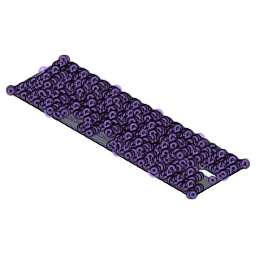
top_layout v3 (Autodesk Fusion 360 design; units mm, degrees)
Autodesk Fusion 360 part; units mm, degrees
(part 1 of 8)
sketch "Sketch2" plane through (0, 0, 0) normal (0, 0, 1) x (1, 0, 0)
  line L0 (124.062, 16.7831) -> (124.062, 15.7827)
  line L1 (124.062, 15.7827) -> (123.263, 15.7827)
  line L2 (123.263, 15.7827) -> (123.263, 12.6848)
  line L3 (123.263, 12.6848) -> (124.062, 12.6848)
  line L4 (124.062, 12.6848) -> (124.062, 12.0826)
  line L5 (124.062, 12.0826) -> (84.4381, 12.0826)
  line L6 (84.4381, 12.0826) -> (84.4381, 15.3128)
  line L7 (84.4381, 15.3128) -> (77.687, 15.3128)
  line L8 (77.687, 15.3128) -> (77.687, 12.0826)
  line L9 (77.687, 12.0826) -> (76.8629, 12.0826)
  line L10 (76.8629, 12.0826) -> (76.8629, 9.2838)
  line L11 (76.8629, 9.2838) -> (77.687, 9.2838)
  line L12 (77.687, 9.2838) -> (77.687, 3.0138)
  line L13 (77.687, 3.0138) -> (79.412, 3.0138)
  line L14 (79.412, 3.0138) -> (79.412, 1.8135)
  line L15 (79.412, 1.8135) -> (82.7126, 1.8135)
  line L16 (82.7126, 1.8135) -> (82.7126, 3.0138)
  line L17 (82.7126, 3.0138) -> (84.4381, 3.0138)
  line L18 (84.4381, 3.0138) -> (84.4381, 7.4841)
  line L19 (84.4381, 7.4841) -> (124.062, 7.4841)
  line L20 (124.062, 7.4841) -> (124.062, 6.8833)
  line L21 (124.062, 6.8833) -> (123.263, 6.8833)
  line L22 (123.263, 6.8833) -> (123.263, 3.7827)
  line L23 (123.263, 3.7827) -> (124.062, 3.7827)
  line L24 (124.062, 3.7827) -> (124.062, 2.7836)
  line L25 (124.062, 2.7836) -> (138.063, 2.7836)
  line L26 (138.063, 2.7836) -> (138.063, 3.7827)
  line L27 (138.063, 3.7827) -> (138.862, 3.7827)
  line L28 (138.862, 3.7827) -> (138.862, 6.8833)
  line L29 (138.862, 6.8833) -> (138.063, 6.8833)
  line L30 (138.063, 6.8833) -> (138.063, 7.4841)
  line L31 (138.063, 7.4841) -> (177.687, 7.4841)
  line L32 (177.687, 7.4841) -> (177.687, 3.0138)
  line L33 (177.687, 3.0138) -> (179.412, 3.0138)
  line L34 (179.412, 3.0138) -> (179.412, 1.8135)
  line L35 (179.412, 1.8135) -> (182.713, 1.8135)
  line L36 (182.713, 1.8135) -> (182.713, 3.0138)
  line L37 (182.713, 3.0138) -> (184.438, 3.0138)
  line L38 (184.438, 3.0138) -> (184.438, 9.2838)
  line L39 (184.438, 9.2838) -> (185.262, 9.2838)
  line L40 (185.262, 9.2838) -> (185.262, 12.0826)
  line L41 (185.262, 12.0826) -> (184.438, 12.0826)
  line L42 (184.438, 12.0826) -> (184.438, 15.3128)
  line L43 (184.438, 15.3128) -> (177.687, 15.3128)
  line L44 (177.687, 15.3128) -> (177.687, 12.0826)
  line L45 (177.687, 12.0826) -> (138.063, 12.0826)
  line L46 (138.063, 12.0826) -> (138.063, 12.6848)
  line L47 (138.063, 12.6848) -> (138.862, 12.6848)
  line L48 (138.862, 12.6848) -> (138.862, 15.7827)
  line L49 (138.862, 15.7827) -> (138.063, 15.7827)
  line L50 (138.063, 15.7827) -> (138.063, 16.7831)
  line L51 (138.063, 16.7831) -> (124.062, 16.7831)
  line L52 (5.0009, 16.7831) -> (5.0009, 15.7827)
  line L53 (5.0009, 15.7827) -> (4.2003, 15.7827)
  line L54 (4.2003, 15.7827) -> (4.2003, 12.6848)
  line L55 (4.2003, 12.6848) -> (5.0009, 12.6848)
  line L56 (5.0009, 12.6848) -> (5.0009, 6.8833)
  line L57 (5.0009, 6.8833) -> (4.2003, 6.8833)
  line L58 (4.2003, 6.8833) -> (4.2003, 3.7827)
  line L59 (4.2003, 3.7827) -> (5.0009, 3.7827)
  line L60 (5.0009, 3.7827) -> (5.0009, 2.7836)
  line L61 (5.0009, 2.7836) -> (19.0004, 2.7836)
  line L62 (19.0004, 2.7836) -> (19.0004, 3.7827)
  line L63 (19.0004, 3.7827) -> (19.801, 3.7827)
  line L64 (19.801, 3.7827) -> (19.801, 6.8833)
  line L65 (19.801, 6.8833) -> (19.0004, 6.8833)
  line L66 (19.0004, 6.8833) -> (19.0004, 12.6848)
  line L67 (19.0004, 12.6848) -> (19.801, 12.6848)
  line L68 (19.801, 12.6848) -> (19.801, 15.7827)
  line L69 (19.801, 15.7827) -> (19.0004, 15.7827)
  line L70 (19.0004, 15.7827) -> (19.0004, 16.7831)
  line L71 (19.0004, 16.7831) -> (5.0009, 16.7831)
  line L72 (28.812, 16.7831) -> (28.812, 15.7827)
  line L73 (28.812, 15.7827) -> (28.0128, 15.7827)
  line L74 (28.0128, 15.7827) -> (28.0128, 12.6848)
  line L75 (28.0128, 12.6848) -> (28.812, 12.6848)
  line L76 (28.812, 12.6848) -> (28.812, 6.8833)
  line L77 (28.812, 6.8833) -> (28.0128, 6.8833)
  line L78 (28.0128, 6.8833) -> (28.0128, 3.7827)
  line L79 (28.0128, 3.7827) -> (28.812, 3.7827)
  line L80 (28.812, 3.7827) -> (28.812, 2.7836)
  line L81 (28.812, 2.7836) -> (42.8128, 2.7836)
  line L82 (42.8128, 2.7836) -> (42.8128, 3.7827)
  line L83 (42.8128, 3.7827) -> (43.6122, 3.7827)
  line L84 (43.6122, 3.7827) -> (43.6122, 6.8833)
  line L85 (43.6122, 6.8833) -> (42.8128, 6.8833)
  line L86 (42.8128, 6.8833) -> (42.8128, 12.6848)
  line L87 (42.8128, 12.6848) -> (43.6122, 12.6848)
  line L88 (43.6122, 12.6848) -> (43.6122, 15.7827)
  line L89 (43.6122, 15.7827) -> (42.8128, 15.7827)
  line L90 (42.8128, 15.7827) -> (42.8128, 16.7831)
  line L91 (42.8128, 16.7831) -> (28.812, 16.7831)
  line L92 (52.626, 16.7831) -> (52.626, 15.7827)
  line L93 (52.626, 15.7827) -> (51.8252, 15.7827)
  line L94 (51.8252, 15.7827) -> (51.8252, 12.6848)
  line L95 (51.8252, 12.6848) -> (52.626, 12.6848)
  line L96 (52.626, 12.6848) -> (52.626, 6.8833)
  line L97 (52.626, 6.8833) -> (51.8252, 6.8833)
  line L98 (51.8252, 6.8833) -> (51.8252, 3.7827)
  line L99 (51.8252, 3.7827) -> (52.626, 3.7827)
  line L100 (52.626, 3.7827) -> (52.626, 2.7836)
  line L101 (52.626, 2.7836) -> (66.6253, 2.7836)
  line L102 (66.6253, 2.7836) -> (66.6253, 3.7827)
  line L103 (66.6253, 3.7827) -> (67.4261, 3.7827)
  line L104 (67.4261, 3.7827) -> (67.4261, 6.8833)
  line L105 (67.4261, 6.8833) -> (66.6253, 6.8833)
  line L106 (66.6253, 6.8833) -> (66.6253, 12.6848)
  line L107 (66.6253, 12.6848) -> (67.4261, 12.6848)
  line L108 (67.4261, 12.6848) -> (67.4261, 15.7827)
  line L109 (67.4261, 15.7827) -> (66.6253, 15.7827)
  line L110 (66.6253, 15.7827) -> (66.6253, 16.7831)
  line L111 (66.6253, 16.7831) -> (52.626, 16.7831)
  line L112 (195.501, 16.7831) -> (195.501, 15.7827)
  line L113 (195.501, 15.7827) -> (194.7, 15.7827)
  line L114 (194.7, 15.7827) -> (194.7, 12.6848)
  line L115 (194.7, 12.6848) -> (195.501, 12.6848)
  line L116 (195.501, 12.6848) -> (195.501, 6.8833)
  line L117 (195.501, 6.8833) -> (194.7, 6.8833)
  line L118 (194.7, 6.8833) -> (194.7, 3.7827)
  line L119 (194.7, 3.7827) -> (195.501, 3.7827)
  line L120 (195.501, 3.7827) -> (195.501, 2.7836)
  line L121 (195.501, 2.7836) -> (209.5, 2.7836)
  line L122 (209.5, 2.7836) -> (209.5, 3.7827)
  line L123 (209.5, 3.7827) -> (210.301, 3.7827)
  line L124 (210.301, 3.7827) -> (210.301, 6.8833)
  line L125 (210.301, 6.8833) -> (209.5, 6.8833)
  line L126 (209.5, 6.8833) -> (209.5, 12.6848)
  line L127 (209.5, 12.6848) -> (210.301, 12.6848)
  line L128 (210.301, 12.6848) -> (210.301, 15.7827)
  line L129 (210.301, 15.7827) -> (209.5, 15.7827)
  line L130 (209.5, 15.7827) -> (209.5, 16.7831)
  line L131 (209.5, 16.7831) -> (195.501, 16.7831)
  line L132 (219.312, 16.7831) -> (219.312, 15.7827)
  line L133 (219.312, 15.7827) -> (218.513, 15.7827)
  line L134 (218.513, 15.7827) -> (218.513, 12.6848)
  line L135 (218.513, 12.6848) -> (219.312, 12.6848)
  line L136 (219.312, 12.6848) -> (219.312, 6.8833)
  line L137 (219.312, 6.8833) -> (218.513, 6.8833)
  line L138 (218.513, 6.8833) -> (218.513, 3.7827)
  line L139 (218.513, 3.7827) -> (219.312, 3.7827)
  line L140 (219.312, 3.7827) -> (219.312, 2.7836)
  line L141 (219.312, 2.7836) -> (233.313, 2.7836)
  line L142 (233.313, 2.7836) -> (233.313, 3.7827)
  line L143 (233.313, 3.7827) -> (234.112, 3.7827)
  line L144 (234.112, 3.7827) -> (234.112, 6.8833)
  line L145 (234.112, 6.8833) -> (233.313, 6.8833)
  line L146 (233.313, 6.8833) -> (233.313, 12.6848)
  line L147 (233.313, 12.6848) -> (234.112, 12.6848)
  line L148 (234.112, 12.6848) -> (234.112, 15.7827)
  line L149 (234.112, 15.7827) -> (233.313, 15.7827)
  line L150 (233.313, 15.7827) -> (233.313, 16.7831)
  line L151 (233.313, 16.7831) -> (219.312, 16.7831)
  line L152 (243.126, 16.7831) -> (243.126, 15.7827)
  line L153 (243.126, 15.7827) -> (242.325, 15.7827)
  line L154 (242.325, 15.7827) -> (242.325, 12.6848)
  line L155 (242.325, 12.6848) -> (243.126, 12.6848)
  line L156 (243.126, 12.6848) -> (243.126, 6.8833)
  line L157 (243.126, 6.8833) -> (242.325, 6.8833)
  line L158 (242.325, 6.8833) -> (242.325, 3.7827)
  line L159 (242.325, 3.7827) -> (243.126, 3.7827)
  line L160 (243.126, 3.7827) -> (243.126, 2.7836)
  line L161 (243.126, 2.7836) -> (257.125, 2.7836)
  line L162 (257.125, 2.7836) -> (257.125, 3.7827)
  line L163 (257.125, 3.7827) -> (257.926, 3.7827)
  line L164 (257.926, 3.7827) -> (257.926, 6.8833)
  line L165 (257.926, 6.8833) -> (257.125, 6.8833)
  line L166 (257.125, 6.8833) -> (257.125, 12.6848)
  line L167 (257.125, 12.6848) -> (257.926, 12.6848)
  line L168 (257.926, 12.6848) -> (257.926, 15.7827)
  line L169 (257.926, 15.7827) -> (257.125, 15.7827)
  line L170 (257.125, 15.7827) -> (257.125, 16.7831)
  line L171 (257.125, 16.7831) -> (243.126, 16.7831)
  line L172 (274.082, 16.7831) -> (274.082, 15.7827)
  line L173 (274.082, 15.7827) -> (273.281, 15.7827)
  line L174 (273.281, 15.7827) -> (273.281, 12.6848)
  line L175 (273.281, 12.6848) -> (274.082, 12.6848)
  line L176 (274.082, 12.6848) -> (274.082, 6.8833)
  line L177 (274.082, 6.8833) -> (273.281, 6.8833)
  line L178 (273.281, 6.8833) -> (273.281, 3.7827)
  line L179 (273.281, 3.7827) -> (274.082, 3.7827)
  line L180 (274.082, 3.7827) -> (274.082, 2.7836)
  line L181 (274.082, 2.7836) -> (288.082, 2.7836)
  line L182 (288.082, 2.7836) -> (288.082, 3.7827)
  line L183 (288.082, 3.7827) -> (288.881, 3.7827)
  line L184 (288.881, 3.7827) -> (288.881, 6.8833)
  line L185 (288.881, 6.8833) -> (288.082, 6.8833)
  line L186 (288.082, 6.8833) -> (288.082, 12.6848)
  line L187 (288.082, 12.6848) -> (288.881, 12.6848)
  line L188 (288.881, 12.6848) -> (288.881, 15.7827)
  line L189 (288.881, 15.7827) -> (288.082, 15.7827)
  line L190 (288.082, 15.7827) -> (288.082, 16.7831)
  line L191 (288.082, 16.7831) -> (274.082, 16.7831)
  line L192 (293.132, 16.7831) -> (293.132, 15.7827)
  line L193 (293.132, 15.7827) -> (292.331, 15.7827)
  line L194 (292.331, 15.7827) -> (292.331, 12.6848)
  line L195 (292.331, 12.6848) -> (293.132, 12.6848)
  line L196 (293.132, 12.6848) -> (293.132, 6.8833)
  line L197 (293.132, 6.8833) -> (292.331, 6.8833)
  line L198 (292.331, 6.8833) -> (292.331, 3.7827)
  line L199 (292.331, 3.7827) -> (293.132, 3.7827)
  line L200 (293.132, 3.7827) -> (293.132, 2.7836)
  line L201 (293.132, 2.7836) -> (307.132, 2.7836)
  line L202 (307.132, 2.7836) -> (307.132, 3.7827)
  line L203 (307.132, 3.7827) -> (307.931, 3.7827)
  line L204 (307.931, 3.7827) -> (307.931, 6.8833)
  line L205 (307.931, 6.8833) -> (307.132, 6.8833)
  line L206 (307.132, 6.8833) -> (307.132, 12.6848)
  line L207 (307.132, 12.6848) -> (307.931, 12.6848)
  line L208 (307.931, 12.6848) -> (307.931, 15.7827)
  line L209 (307.931, 15.7827) -> (307.132, 15.7827)
  line L210 (307.132, 15.7827) -> (307.132, 16.7831)
  line L211 (307.132, 16.7831) -> (293.132, 16.7831)
  line L212 (312.182, 16.7831) -> (312.182, 15.7827)
  line L213 (312.182, 15.7827) -> (311.381, 15.7827)
  line L214 (311.381, 15.7827) -> (311.381, 12.6848)
  line L215 (311.381, 12.6848) -> (312.182, 12.6848)
  line L216 (312.182, 12.6848) -> (312.182, 6.8833)
  line L217 (312.182, 6.8833) -> (311.381, 6.8833)
  line L218 (311.381, 6.8833) -> (311.381, 3.7827)
  line L219 (311.381, 3.7827) -> (312.182, 3.7827)
  line L220 (312.182, 3.7827) -> (312.182, 2.7836)
  line L221 (312.182, 2.7836) -> (326.182, 2.7836)
  line L222 (326.182, 2.7836) -> (326.182, 3.7827)
  line L223 (326.182, 3.7827) -> (326.981, 3.7827)
  line L224 (326.981, 3.7827) -> (326.981, 6.8833)
  line L225 (326.981, 6.8833) -> (326.182, 6.8833)
  line L226 (326.182, 6.8833) -> (326.182, 12.6848)
  line L227 (326.182, 12.6848) -> (326.981, 12.6848)
  line L228 (326.981, 12.6848) -> (326.981, 15.7827)
  line L229 (326.981, 15.7827) -> (326.182, 15.7827)
  line L230 (326.182, 15.7827) -> (326.182, 16.7831)
  line L231 (326.182, 16.7831) -> (312.182, 16.7831)
  line L232 (14.5259, 35.833) -> (14.5259, 34.8327)
  line L233 (14.5259, 34.8327) -> (13.7253, 34.8327)
  line L234 (13.7253, 34.8327) -> (13.7253, 31.7348)
  line L235 (13.7253, 31.7348) -> (14.5259, 31.7348)
  line L236 (14.5259, 31.7348) -> (14.5259, 31.1326)
  line L237 (14.5259, 31.1326) -> (13.0004, 31.1326)
  line L238 (13.0004, 31.1326) -> (13.0004, 34.3628)
  line L239 (13.0004, 34.3628) -> (6.2508, 34.3628)
  line L240 (6.2508, 34.3628) -> (6.2508, 31.1326)
  line L241 (6.2508, 31.1326) -> (5.4253, 31.1326)
  line L242 (5.4253, 31.1326) -> (5.4253, 28.3338)
  line L243 (5.4253, 28.3338) -> (6.2508, 28.3338)
  line L244 (6.2508, 28.3338) -> (6.2508, 22.0638)
  line L245 (6.2508, 22.0638) -> (7.9761, 22.0638)
  line L246 (7.9761, 22.0638) -> (7.9761, 20.8635)
  line L247 (7.9761, 20.8635) -> (11.2751, 20.8635)
  line L248 (11.2751, 20.8635) -> (11.2751, 22.0638)
  line L249 (11.2751, 22.0638) -> (13.0004, 22.0638)
  line L250 (13.0004, 22.0638) -> (13.0004, 26.5327)
  line L251 (13.0004, 26.5327) -> (14.5259, 26.5327)
  line L252 (14.5259, 26.5327) -> (14.5259, 25.9333)
  line L253 (14.5259, 25.9333) -> (13.7253, 25.9333)
  line L254 (13.7253, 25.9333) -> (13.7253, 22.8327)
  line L255 (13.7253, 22.8327) -> (14.5259, 22.8327)
  line L256 (14.5259, 22.8327) -> (14.5259, 21.8336)
  line L257 (14.5259, 21.8336) -> (28.5254, 21.8336)
  line L258 (28.5254, 21.8336) -> (28.5254, 22.8327)
  line L259 (28.5254, 22.8327) -> (29.326, 22.8327)
  line L260 (29.326, 22.8327) -> (29.326, 25.9333)
  line L261 (29.326, 25.9333) -> (28.5254, 25.9333)
  line L262 (28.5254, 25.9333) -> (28.5254, 26.5327)
  line L263 (28.5254, 26.5327) -> (30.0509, 26.5327)
  line L264 (30.0509, 26.5327) -> (30.0509, 22.0638)
  line L265 (30.0509, 22.0638) -> (31.7748, 22.0638)
  line L266 (31.7748, 22.0638) -> (31.7748, 20.8635)
  line L267 (31.7748, 20.8635) -> (35.0752, 20.8635)
  line L268 (35.0752, 20.8635) -> (35.0752, 22.0638)
  line L269 (35.0752, 22.0638) -> (36.8004, 22.0638)
  line L270 (36.8004, 22.0638) -> (36.8004, 28.3338)
  line L271 (36.8004, 28.3338) -> (37.6259, 28.3338)
  line L272 (37.6259, 28.3338) -> (37.6259, 31.1326)
  line L273 (37.6259, 31.1326) -> (36.8004, 31.1326)
  line L274 (36.8004, 31.1326) -> (36.8004, 34.3628)
  line L275 (36.8004, 34.3628) -> (30.0509, 34.3628)
  line L276 (30.0509, 34.3628) -> (30.0509, 31.1326)
  line L277 (30.0509, 31.1326) -> (28.5254, 31.1326)
  line L278 (28.5254, 31.1326) -> (28.5254, 31.7348)
  line L279 (28.5254, 31.7348) -> (29.326, 31.7348)
  line L280 (29.326, 31.7348) -> (29.326, 34.8327)
  line L281 (29.326, 34.8327) -> (28.5254, 34.8327)
  line L282 (28.5254, 34.8327) -> (28.5254, 35.833)
  line L283 (28.5254, 35.833) -> (14.5259, 35.833)
  line L284 (252.65, 35.833) -> (252.65, 34.8327)
  line L285 (252.65, 34.8327) -> (251.849, 34.8327)
  line L286 (251.849, 34.8327) -> (251.849, 31.7348)
  line L287 (251.849, 31.7348) -> (252.65, 31.7348)
  line L288 (252.65, 31.7348) -> (252.65, 31.1326)
  line L289 (252.65, 31.1326) -> (251.126, 31.1326)
  line L290 (251.126, 31.1326) -> (251.126, 34.3628)
  line L291 (251.126, 34.3628) -> (244.376, 34.3628)
  line L292 (244.376, 34.3628) -> (244.376, 31.1326)
  line L293 (244.376, 31.1326) -> (243.55, 31.1326)
  line L294 (243.55, 31.1326) -> (243.55, 28.3338)
  line L295 (243.55, 28.3338) -> (244.376, 28.3338)
  line L296 (244.376, 28.3338) -> (244.376, 22.0638)
  line L297 (244.376, 22.0638) -> (246.101, 22.0638)
  line L298 (246.101, 22.0638) -> (246.101, 20.8635)
  line L299 (246.101, 20.8635) -> (249.4, 20.8635)
  line L300 (249.4, 20.8635) -> (249.4, 22.0638)
  line L301 (249.4, 22.0638) -> (251.126, 22.0638)
  line L302 (251.126, 22.0638) -> (251.126, 26.5327)
  line L303 (251.126, 26.5327) -> (252.65, 26.5327)
  line L304 (252.65, 26.5327) -> (252.65, 25.9333)
  line L305 (252.65, 25.9333) -> (251.849, 25.9333)
  line L306 (251.849, 25.9333) -> (251.849, 22.8327)
  line L307 (251.849, 22.8327) -> (252.65, 22.8327)
  line L308 (252.65, 22.8327) -> (252.65, 21.8336)
  line L309 (252.65, 21.8336) -> (266.65, 21.8336)
  line L310 (266.65, 21.8336) -> (266.65, 22.8327)
  line L311 (266.65, 22.8327) -> (267.451, 22.8327)
  line L312 (267.451, 22.8327) -> (267.451, 25.9333)
  line L313 (267.451, 25.9333) -> (266.65, 25.9333)
  line L314 (266.65, 25.9333) -> (266.65, 26.5327)
  line L315 (266.65, 26.5327) -> (268.176, 26.5327)
  line L316 (268.176, 26.5327) -> (268.176, 22.0638)
  line L317 (268.176, 22.0638) -> (269.9, 22.0638)
  line L318 (269.9, 22.0638) -> (269.9, 20.8635)
  line L319 (269.9, 20.8635) -> (273.2, 20.8635)
  line L320 (273.2, 20.8635) -> (273.2, 22.0638)
  line L321 (273.2, 22.0638) -> (274.925, 22.0638)
  line L322 (274.925, 22.0638) -> (274.925, 28.3338)
  line L323 (274.925, 28.3338) -> (275.751, 28.3338)
  line L324 (275.751, 28.3338) -> (275.751, 31.1326)
  line L325 (275.751, 31.1326) -> (274.925, 31.1326)
  line L326 (274.925, 31.1326) -> (274.925, 34.3628)
  line L327 (274.925, 34.3628) -> (268.176, 34.3628)
  line L328 (268.176, 34.3628) -> (268.176, 31.1326)
  line L329 (268.176, 31.1326) -> (266.65, 31.1326)
  line L330 (266.65, 31.1326) -> (266.65, 31.7348)
  line L331 (266.65, 31.7348) -> (267.451, 31.7348)
  line L332 (267.451, 31.7348) -> (267.451, 34.8327)
  line L333 (267.451, 34.8327) -> (266.65, 34.8327)
  line L334 (266.65, 34.8327) -> (266.65, 35.833)
  line L335 (266.65, 35.833) -> (252.65, 35.833)
  line L336 (45.4822, 35.833) -> (45.4822, 34.8327)
  line L337 (45.4822, 34.8327) -> (44.6814, 34.8327)
  line L338 (44.6814, 34.8327) -> (44.6814, 31.7348)
  line L339 (44.6814, 31.7348) -> (45.4822, 31.7348)
  line L340 (45.4822, 31.7348) -> (45.4822, 25.9333)
  line L341 (45.4822, 25.9333) -> (44.6814, 25.9333)
  line L342 (44.6814, 25.9333) -> (44.6814, 22.8327)
  line L343 (44.6814, 22.8327) -> (45.4822, 22.8327)
  line L344 (45.4822, 22.8327) -> (45.4822, 21.8336)
  line L345 (45.4822, 21.8336) -> (59.4815, 21.8336)
  line L346 (59.4815, 21.8336) -> (59.4815, 22.8327)
  line L347 (59.4815, 22.8327) -> (60.2809, 22.8327)
  line L348 (60.2809, 22.8327) -> (60.2809, 25.9333)
  line L349 (60.2809, 25.9333) -> (59.4815, 25.9333)
  line L350 (59.4815, 25.9333) -> (59.4815, 31.7348)
  line L351 (59.4815, 31.7348) -> (60.2809, 31.7348)
  line L352 (60.2809, 31.7348) -> (60.2809, 34.8327)
  line L353 (60.2809, 34.8327) -> (59.4815, 34.8327)
  line L354 (59.4815, 34.8327) -> (59.4815, 35.833)
  line L355 (59.4815, 35.833) -> (45.4822, 35.833)
  line L356 (64.5322, 35.833) -> (64.5322, 34.8327)
  line L357 (64.5322, 34.8327) -> (63.7314, 34.8327)
  line L358 (63.7314, 34.8327) -> (63.7314, 31.7348)
  line L359 (63.7314, 31.7348) -> (64.5322, 31.7348)
  line L360 (64.5322, 31.7348) -> (64.5322, 25.9333)
  line L361 (64.5322, 25.9333) -> (63.7314, 25.9333)
  line L362 (63.7314, 25.9333) -> (63.7314, 22.8327)
  line L363 (63.7314, 22.8327) -> (64.5322, 22.8327)
  line L364 (64.5322, 22.8327) -> (64.5322, 21.8336)
  line L365 (64.5322, 21.8336) -> (78.5315, 21.8336)
  line L366 (78.5315, 21.8336) -> (78.5315, 22.8327)
  line L367 (78.5315, 22.8327) -> (79.3309, 22.8327)
  line L368 (79.3309, 22.8327) -> (79.3309, 25.9333)
  line L369 (79.3309, 25.9333) -> (78.5315, 25.9333)
  line L370 (78.5315, 25.9333) -> (78.5315, 31.7348)
  line L371 (78.5315, 31.7348) -> (79.3309, 31.7348)
  line L372 (79.3309, 31.7348) -> (79.3309, 34.8327)
  line L373 (79.3309, 34.8327) -> (78.5315, 34.8327)
  line L374 (78.5315, 34.8327) -> (78.5315, 35.833)
  line L375 (78.5315, 35.833) -> (64.5322, 35.833)
  line L376 (83.5822, 35.833) -> (83.5822, 34.8327)
  line L377 (83.5822, 34.8327) -> (82.7814, 34.8327)
  line L378 (82.7814, 34.8327) -> (82.7814, 31.7348)
  line L379 (82.7814, 31.7348) -> (83.5822, 31.7348)
  line L380 (83.5822, 31.7348) -> (83.5822, 25.9333)
  line L381 (83.5822, 25.9333) -> (82.7814, 25.9333)
  line L382 (82.7814, 25.9333) -> (82.7814, 22.8327)
  line L383 (82.7814, 22.8327) -> (83.5822, 22.8327)
  line L384 (83.5822, 22.8327) -> (83.5822, 21.8336)
  line L385 (83.5822, 21.8336) -> (97.5815, 21.8336)
  line L386 (97.5815, 21.8336) -> (97.5815, 22.8327)
  line L387 (97.5815, 22.8327) -> (98.3809, 22.8327)
  line L388 (98.3809, 22.8327) -> (98.3809, 25.9333)
  line L389 (98.3809, 25.9333) -> (97.5815, 25.9333)
  line L390 (97.5815, 25.9333) -> (97.5815, 31.7348)
  line L391 (97.5815, 31.7348) -> (98.3809, 31.7348)
  line L392 (98.3809, 31.7348) -> (98.3809, 34.8327)
  line L393 (98.3809, 34.8327) -> (97.5815, 34.8327)
  line L394 (97.5815, 34.8327) -> (97.5815, 35.833)
  line L395 (97.5815, 35.833) -> (83.5822, 35.833)
  line L396 (102.632, 35.833) -> (102.632, 34.8327)
  line L397 (102.632, 34.8327) -> (101.831, 34.8327)
  line L398 (101.831, 34.8327) -> (101.831, 31.7348)
  line L399 (101.831, 31.7348) -> (102.632, 31.7348)
  line L400 (102.632, 31.7348) -> (102.632, 25.9333)
  line L401 (102.632, 25.9333) -> (101.831, 25.9333)
  line L402 (101.831, 25.9333) -> (101.831, 22.8327)
  line L403 (101.831, 22.8327) -> (102.632, 22.8327)
  line L404 (102.632, 22.8327) -> (102.632, 21.8336)
  line L405 (102.632, 21.8336) -> (116.632, 21.8336)
  line L406 (116.632, 21.8336) -> (116.632, 22.8327)
  line L407 (116.632, 22.8327) -> (117.431, 22.8327)
  line L408 (117.431, 22.8327) -> (117.431, 25.9333)
  line L409 (117.431, 25.9333) -> (116.632, 25.9333)
  line L410 (116.632, 25.9333) -> (116.632, 31.7348)
  line L411 (116.632, 31.7348) -> (117.431, 31.7348)
  line L412 (117.431, 31.7348) -> (117.431, 34.8327)
  line L413 (117.431, 34.8327) -> (116.632, 34.8327)
  line L414 (116.632, 34.8327) -> (116.632, 35.833)
  line L415 (116.632, 35.833) -> (102.632, 35.833)
  line L416 (121.682, 35.833) -> (121.682, 34.8327)
  line L417 (121.682, 34.8327) -> (120.881, 34.8327)
  line L418 (120.881, 34.8327) -> (120.881, 31.7348)
  line L419 (120.881, 31.7348) -> (121.682, 31.7348)
  line L420 (121.682, 31.7348) -> (121.682, 25.9333)
  line L421 (121.682, 25.9333) -> (120.881, 25.9333)
  line L422 (120.881, 25.9333) -> (120.881, 22.8327)
  line L423 (120.881, 22.8327) -> (121.682, 22.8327)
  line L424 (121.682, 22.8327) -> (121.682, 21.8336)
  line L425 (121.682, 21.8336) -> (135.682, 21.8336)
  line L426 (135.682, 21.8336) -> (135.682, 22.8327)
  line L427 (135.682, 22.8327) -> (136.481, 22.8327)
  line L428 (136.481, 22.8327) -> (136.481, 25.9333)
  line L429 (136.481, 25.9333) -> (135.682, 25.9333)
  line L430 (135.682, 25.9333) -> (135.682, 31.7348)
  line L431 (135.682, 31.7348) -> (136.481, 31.7348)
  line L432 (136.481, 31.7348) -> (136.481, 34.8327)
  line L433 (136.481, 34.8327) -> (135.682, 34.8327)
  line L434 (135.682, 34.8327) -> (135.682, 35.833)
  line L435 (135.682, 35.833) -> (121.682, 35.833)
  line L436 (140.732, 35.833) -> (140.732, 34.8327)
  line L437 (140.732, 34.8327) -> (139.931, 34.8327)
  line L438 (139.931, 34.8327) -> (139.931, 31.7348)
  line L439 (139.931, 31.7348) -> (140.732, 31.7348)
  line L440 (140.732, 31.7348) -> (140.732, 25.9333)
  line L441 (140.732, 25.9333) -> (139.931, 25.9333)
  line L442 (139.931, 25.9333) -> (139.931, 22.8327)
  line L443 (139.931, 22.8327) -> (140.732, 22.8327)
  line L444 (140.732, 22.8327) -> (140.732, 21.8336)
  line L445 (140.732, 21.8336) -> (154.732, 21.8336)
  line L446 (154.732, 21.8336) -> (154.732, 22.8327)
  line L447 (154.732, 22.8327) -> (155.531, 22.8327)
  line L448 (155.531, 22.8327) -> (155.531, 25.9333)
  line L449 (155.531, 25.9333) -> (154.732, 25.9333)
  line L450 (154.732, 25.9333) -> (154.732, 31.7348)
  line L451 (154.732, 31.7348) -> (155.531, 31.7348)
  line L452 (155.531, 31.7348) -> (155.531, 34.8327)
  line L453 (155.531, 34.8327) -> (154.732, 34.8327)
  line L454 (154.732, 34.8327) -> (154.732, 35.833)
  line L455 (154.732, 35.833) -> (140.732, 35.833)
  line L456 (159.782, 35.833) -> (159.782, 34.8327)
  line L457 (159.782, 34.8327) -> (158.981, 34.8327)
  line L458 (158.981, 34.8327) -> (158.981, 31.7348)
  line L459 (158.981, 31.7348) -> (159.782, 31.7348)
  line L460 (159.782, 31.7348) -> (159.782, 25.9333)
  line L461 (159.782, 25.9333) -> (158.981, 25.9333)
  line L462 (158.981, 25.9333) -> (158.981, 22.8327)
  line L463 (158.981, 22.8327) -> (159.782, 22.8327)
  line L464 (159.782, 22.8327) -> (159.782, 21.8336)
  line L465 (159.782, 21.8336) -> (173.782, 21.8336)
  line L466 (173.782, 21.8336) -> (173.782, 22.8327)
  line L467 (173.782, 22.8327) -> (174.581, 22.8327)
  line L468 (174.581, 22.8327) -> (174.581, 25.9333)
  line L469 (174.581, 25.9333) -> (173.782, 25.9333)
  line L470 (173.782, 25.9333) -> (173.782, 31.7348)
  line L471 (173.782, 31.7348) -> (174.581, 31.7348)
  line L472 (174.581, 31.7348) -> (174.581, 34.8327)
  line L473 (174.581, 34.8327) -> (173.782, 34.8327)
  line L474 (173.782, 34.8327) -> (173.782, 35.833)
  line L475 (173.782, 35.833) -> (159.782, 35.833)
  line L476 (178.832, 35.833) -> (178.832, 34.8327)
  line L477 (178.832, 34.8327) -> (178.031, 34.8327)
  line L478 (178.031, 34.8327) -> (178.031, 31.7348)
  line L479 (178.031, 31.7348) -> (178.832, 31.7348)
  line L480 (178.832, 31.7348) -> (178.832, 25.9333)
  line L481 (178.832, 25.9333) -> (178.031, 25.9333)
  line L482 (178.031, 25.9333) -> (178.031, 22.8327)
  line L483 (178.031, 22.8327) -> (178.832, 22.8327)
  line L484 (178.832, 22.8327) -> (178.832, 21.8336)
  line L485 (178.832, 21.8336) -> (192.832, 21.8336)
  line L486 (192.832, 21.8336) -> (192.832, 22.8327)
  line L487 (192.832, 22.8327) -> (193.631, 22.8327)
  line L488 (193.631, 22.8327) -> (193.631, 25.9333)
  line L489 (193.631, 25.9333) -> (192.832, 25.9333)
  line L490 (192.832, 25.9333) -> (192.832, 31.7348)
  line L491 (192.832, 31.7348) -> (193.631, 31.7348)
  line L492 (193.631, 31.7348) -> (193.631, 34.8327)
  line L493 (193.631, 34.8327) -> (192.832, 34.8327)
  line L494 (192.832, 34.8327) -> (192.832, 35.833)
  line L495 (192.832, 35.833) -> (178.832, 35.833)
  line L496 (197.882, 35.833) -> (197.882, 34.8327)
  line L497 (197.882, 34.8327) -> (197.081, 34.8327)
  line L498 (197.081, 34.8327) -> (197.081, 31.7348)
  line L499 (197.081, 31.7348) -> (197.882, 31.7348)
  line L500 (197.882, 31.7348) -> (197.882, 25.9333)
  line L501 (197.882, 25.9333) -> (197.081, 25.9333)
  line L502 (197.081, 25.9333) -> (197.081, 22.8327)
  line L503 (197.081, 22.8327) -> (197.882, 22.8327)
  line L504 (197.882, 22.8327) -> (197.882, 21.8336)
  line L505 (197.882, 21.8336) -> (211.882, 21.8336)
  line L506 (211.882, 21.8336) -> (211.882, 22.8327)
  line L507 (211.882, 22.8327) -> (212.681, 22.8327)
  line L508 (212.681, 22.8327) -> (212.681, 25.9333)
  line L509 (212.681, 25.9333) -> (211.882, 25.9333)
  line L510 (211.882, 25.9333) -> (211.882, 31.7348)
  line L511 (211.882, 31.7348) -> (212.681, 31.7348)
  line L512 (212.681, 31.7348) -> (212.681, 34.8327)
  line L513 (212.681, 34.8327) -> (211.882, 34.8327)
  line L514 (211.882, 34.8327) -> (211.882, 35.833)
  line L515 (211.882, 35.833) -> (197.882, 35.833)
  line L516 (216.932, 35.833) -> (216.932, 34.8327)
  line L517 (216.932, 34.8327) -> (216.131, 34.8327)
  line L518 (216.131, 34.8327) -> (216.131, 31.7348)
  line L519 (216.131, 31.7348) -> (216.932, 31.7348)
  line L520 (216.932, 31.7348) -> (216.932, 25.9333)
  line L521 (216.932, 25.9333) -> (216.131, 25.9333)
  line L522 (216.131, 25.9333) -> (216.131, 22.8327)
  line L523 (216.131, 22.8327) -> (216.932, 22.8327)
  line L524 (216.932, 22.8327) -> (216.932, 21.8336)
  line L525 (216.932, 21.8336) -> (230.932, 21.8336)
  line L526 (230.932, 21.8336) -> (230.932, 22.8327)
  line L527 (230.932, 22.8327) -> (231.731, 22.8327)
  line L528 (231.731, 22.8327) -> (231.731, 25.9333)
  line L529 (231.731, 25.9333) -> (230.932, 25.9333)
  line L530 (230.932, 25.9333) -> (230.932, 31.7348)
  line L531 (230.932, 31.7348) -> (231.731, 31.7348)
  line L532 (231.731, 31.7348) -> (231.731, 34.8327)
  line L533 (231.731, 34.8327) -> (230.932, 34.8327)
  line L534 (230.932, 34.8327) -> (230.932, 35.833)
  line L535 (230.932, 35.833) -> (216.932, 35.833)
  line L536 (293.132, 35.833) -> (293.132, 34.8327)
  line L537 (293.132, 34.8327) -> (292.331, 34.8327)
  line L538 (292.331, 34.8327) -> (292.331, 31.7348)
  line L539 (292.331, 31.7348) -> (293.132, 31.7348)
  line L540 (293.132, 31.7348) -> (293.132, 25.9333)
  line L541 (293.132, 25.9333) -> (292.331, 25.9333)
  line L542 (292.331, 25.9333) -> (292.331, 22.8327)
  line L543 (292.331, 22.8327) -> (293.132, 22.8327)
  line L544 (293.132, 22.8327) -> (293.132, 21.8336)
  line L545 (293.132, 21.8336) -> (307.132, 21.8336)
  line L546 (307.132, 21.8336) -> (307.132, 22.8327)
  line L547 (307.132, 22.8327) -> (307.931, 22.8327)
  line L548 (307.931, 22.8327) -> (307.931, 25.9333)
  line L549 (307.931, 25.9333) -> (307.132, 25.9333)
  line L550 (307.132, 25.9333) -> (307.132, 31.7348)
  line L551 (307.132, 31.7348) -> (307.931, 31.7348)
  line L552 (307.931, 31.7348) -> (307.931, 34.8327)
  line L553 (307.931, 34.8327) -> (307.132, 34.8327)
  line L554 (307.132, 34.8327) -> (307.132, 35.833)
  line L555 (307.132, 35.833) -> (293.132, 35.833)
  line L556 (257.412, 54.8831) -> (257.412, 53.8826)
  line L557 (257.412, 53.8826) -> (256.611, 53.8826)
  line L558 (256.611, 53.8826) -> (256.611, 50.7834)
  line L559 (256.611, 50.7834) -> (257.412, 50.7834)
  line L560 (257.412, 50.7834) -> (257.412, 50.1826)
  line L561 (257.412, 50.1826) -> (255.888, 50.1826)
  line L562 (255.888, 50.1826) -> (255.888, 53.4127)
  line L563 (255.888, 53.4127) -> (249.137, 53.4127)
  line L564 (249.137, 53.4127) -> (249.137, 50.1826)
  line L565 (249.137, 50.1826) -> (248.313, 50.1826)
  line L566 (248.313, 50.1826) -> (248.313, 47.3837)
  line L567 (248.313, 47.3837) -> (249.137, 47.3837)
  line L568 (249.137, 47.3837) -> (249.137, 41.1138)
  line L569 (249.137, 41.1138) -> (250.862, 41.1138)
  line L570 (250.862, 41.1138) -> (250.862, 39.9136)
  line L571 (250.862, 39.9136) -> (254.161, 39.9136)
  line L572 (254.161, 39.9136) -> (254.161, 41.1138)
  line L573 (254.161, 41.1138) -> (255.888, 41.1138)
  line L574 (255.888, 41.1138) -> (255.888, 45.5828)
  line L575 (255.888, 45.5828) -> (257.412, 45.5828)
  line L576 (257.412, 45.5828) -> (257.412, 44.9834)
  line L577 (257.412, 44.9834) -> (256.611, 44.9834)
  line L578 (256.611, 44.9834) -> (256.611, 41.8828)
  line L579 (256.611, 41.8828) -> (257.412, 41.8828)
  line L580 (257.412, 41.8828) -> (257.412, 40.8838)
  line L581 (257.412, 40.8838) -> (271.413, 40.8838)
  line L582 (271.413, 40.8838) -> (271.413, 41.8828)
  line L583 (271.413, 41.8828) -> (272.212, 41.8828)
  line L584 (272.212, 41.8828) -> (272.212, 44.9834)
  line L585 (272.212, 44.9834) -> (271.413, 44.9834)
  line L586 (271.413, 44.9834) -> (271.413, 45.5828)
  line L587 (271.413, 45.5828) -> (272.937, 45.5828)
  line L588 (272.937, 45.5828) -> (272.937, 41.1138)
  line L589 (272.937, 41.1138) -> (274.662, 41.1138)
  line L590 (274.662, 41.1138) -> (274.662, 39.9136)
  line L591 (274.662, 39.9136) -> (277.963, 39.9136)
  line L592 (277.963, 39.9136) -> (277.963, 41.1138)
  line L593 (277.963, 41.1138) -> (279.688, 41.1138)
  line L594 (279.688, 41.1138) -> (279.688, 47.3837)
  line L595 (279.688, 47.3837) -> (280.512, 47.3837)
  line L596 (280.512, 47.3837) -> (280.512, 50.1826)
  line L597 (280.512, 50.1826) -> (279.688, 50.1826)
  line L598 (279.688, 50.1826) -> (279.688, 53.4127)
  line L599 (279.688, 53.4127) -> (272.937, 53.4127)
  line L600 (272.937, 53.4127) -> (272.937, 50.1826)
  line L601 (272.937, 50.1826) -> (271.413, 50.1826)
  line L602 (271.413, 50.1826) -> (271.413, 50.7834)
  line L603 (271.413, 50.7834) -> (272.212, 50.7834)
  line L604 (272.212, 50.7834) -> (272.212, 53.8826)
  line L605 (272.212, 53.8826) -> (271.413, 53.8826)
  line L606 (271.413, 53.8826) -> (271.413, 54.8831)
  line L607 (271.413, 54.8831) -> (257.412, 54.8831)
  line L608 (9.762, 54.8831) -> (9.762, 53.8826)
  line L609 (9.762, 53.8826) -> (8.9628, 53.8826)
  line L610 (8.9628, 53.8826) -> (8.9628, 50.7834)
  line L611 (8.9628, 50.7834) -> (9.762, 50.7834)
  line L612 (9.762, 50.7834) -> (9.762, 44.9834)
  line L613 (9.762, 44.9834) -> (8.9628, 44.9834)
  line L614 (8.9628, 44.9834) -> (8.9628, 41.8828)
  line L615 (8.9628, 41.8828) -> (9.762, 41.8828)
  line L616 (9.762, 41.8828) -> (9.762, 40.8838)
  line L617 (9.762, 40.8838) -> (23.7629, 40.8838)
  line L618 (23.7629, 40.8838) -> (23.7629, 41.8828)
  line L619 (23.7629, 41.8828) -> (24.5622, 41.8828)
  line L620 (24.5622, 41.8828) -> (24.5622, 44.9834)
  line L621 (24.5622, 44.9834) -> (23.7629, 44.9834)
  line L622 (23.7629, 44.9834) -> (23.7629, 50.7834)
  line L623 (23.7629, 50.7834) -> (24.5622, 50.7834)
  line L624 (24.5622, 50.7834) -> (24.5622, 53.8826)
  line L625 (24.5622, 53.8826) -> (23.7629, 53.8826)
  line L626 (23.7629, 53.8826) -> (23.7629, 54.8831)
  line L627 (23.7629, 54.8831) -> (9.762, 54.8831)
  line L628 (35.9572, 54.8831) -> (35.9572, 53.8826)
  line L629 (35.9572, 53.8826) -> (35.1565, 53.8826)
  line L630 (35.1565, 53.8826) -> (35.1565, 50.7834)
  line L631 (35.1565, 50.7834) -> (35.9572, 50.7834)
  line L632 (35.9572, 50.7834) -> (35.9572, 44.9834)
  line L633 (35.9572, 44.9834) -> (35.1565, 44.9834)
  line L634 (35.1565, 44.9834) -> (35.1565, 41.8828)
  line L635 (35.1565, 41.8828) -> (35.9572, 41.8828)
  line L636 (35.9572, 41.8828) -> (35.9572, 40.8838)
  line L637 (35.9572, 40.8838) -> (49.9565, 40.8838)
  line L638 (49.9565, 40.8838) -> (49.9565, 41.8828)
  line L639 (49.9565, 41.8828) -> (50.7559, 41.8828)
  line L640 (50.7559, 41.8828) -> (50.7559, 44.9834)
  line L641 (50.7559, 44.9834) -> (49.9565, 44.9834)
  line L642 (49.9565, 44.9834) -> (49.9565, 50.7834)
  line L643 (49.9565, 50.7834) -> (50.7559, 50.7834)
  line L644 (50.7559, 50.7834) -> (50.7559, 53.8826)
  line L645 (50.7559, 53.8826) -> (49.9565, 53.8826)
  line L646 (49.9565, 53.8826) -> (49.9565, 54.8831)
  line L647 (49.9565, 54.8831) -> (35.9572, 54.8831)
  line L648 (55.0072, 54.8831) -> (55.0072, 53.8826)
  line L649 (55.0072, 53.8826) -> (54.2064, 53.8826)
  line L650 (54.2064, 53.8826) -> (54.2064, 50.7834)
  line L651 (54.2064, 50.7834) -> (55.0072, 50.7834)
  line L652 (55.0072, 50.7834) -> (55.0072, 44.9834)
  line L653 (55.0072, 44.9834) -> (54.2064, 44.9834)
  line L654 (54.2064, 44.9834) -> (54.2064, 41.8828)
  line L655 (54.2064, 41.8828) -> (55.0072, 41.8828)
  line L656 (55.0072, 41.8828) -> (55.0072, 40.8838)
  line L657 (55.0072, 40.8838) -> (69.0065, 40.8838)
  line L658 (69.0065, 40.8838) -> (69.0065, 41.8828)
  line L659 (69.0065, 41.8828) -> (69.8059, 41.8828)
  line L660 (69.8059, 41.8828) -> (69.8059, 44.9834)
  line L661 (69.8059, 44.9834) -> (69.0065, 44.9834)
  line L662 (69.0065, 44.9834) -> (69.0065, 50.7834)
  line L663 (69.0065, 50.7834) -> (69.8059, 50.7834)
  line L664 (69.8059, 50.7834) -> (69.8059, 53.8826)
  line L665 (69.8059, 53.8826) -> (69.0065, 53.8826)
  line L666 (69.0065, 53.8826) -> (69.0065, 54.8831)
  line L667 (69.0065, 54.8831) -> (55.0072, 54.8831)
  line L668 (74.0572, 54.8831) -> (74.0572, 53.8826)
  line L669 (74.0572, 53.8826) -> (73.2564, 53.8826)
  line L670 (73.2564, 53.8826) -> (73.2564, 50.7834)
  line L671 (73.2564, 50.7834) -> (74.0572, 50.7834)
  line L672 (74.0572, 50.7834) -> (74.0572, 44.9834)
  line L673 (74.0572, 44.9834) -> (73.2564, 44.9834)
  line L674 (73.2564, 44.9834) -> (73.2564, 41.8828)
  line L675 (73.2564, 41.8828) -> (74.0572, 41.8828)
  line L676 (74.0572, 41.8828) -> (74.0572, 40.8838)
  line L677 (74.0572, 40.8838) -> (88.0565, 40.8838)
  line L678 (88.0565, 40.8838) -> (88.0565, 41.8828)
  line L679 (88.0565, 41.8828) -> (88.8559, 41.8828)
  line L680 (88.8559, 41.8828) -> (88.8559, 44.9834)
  line L681 (88.8559, 44.9834) -> (88.0565, 44.9834)
  line L682 (88.0565, 44.9834) -> (88.0565, 50.7834)
  line L683 (88.0565, 50.7834) -> (88.8559, 50.7834)
  line L684 (88.8559, 50.7834) -> (88.8559, 53.8826)
  line L685 (88.8559, 53.8826) -> (88.0565, 53.8826)
  line L686 (88.0565, 53.8826) -> (88.0565, 54.8831)
  line L687 (88.0565, 54.8831) -> (74.0572, 54.8831)
  line L688 (93.1072, 54.8831) -> (93.1072, 53.8826)
  line L689 (93.1072, 53.8826) -> (92.3064, 53.8826)
  line L690 (92.3064, 53.8826) -> (92.3064, 50.7834)
  line L691 (92.3064, 50.7834) -> (93.1072, 50.7834)
  line L692 (93.1072, 50.7834) -> (93.1072, 44.9834)
  line L693 (93.1072, 44.9834) -> (92.3064, 44.9834)
  line L694 (92.3064, 44.9834) -> (92.3064, 41.8828)
  line L695 (92.3064, 41.8828) -> (93.1072, 41.8828)
  line L696 (93.1072, 41.8828) -> (93.1072, 40.8838)
  line L697 (93.1072, 40.8838) -> (107.107, 40.8838)
  line L698 (107.107, 40.8838) -> (107.107, 41.8828)
  line L699 (107.107, 41.8828) -> (107.906, 41.8828)
  line L700 (107.906, 41.8828) -> (107.906, 44.9834)
  line L701 (107.906, 44.9834) -> (107.107, 44.9834)
  line L702 (107.107, 44.9834) -> (107.107, 50.7834)
  line L703 (107.107, 50.7834) -> (107.906, 50.7834)
  line L704 (107.906, 50.7834) -> (107.906, 53.8826)
  line L705 (107.906, 53.8826) -> (107.107, 53.8826)
  line L706 (107.107, 53.8826) -> (107.107, 54.8831)
  line L707 (107.107, 54.8831) -> (93.1072, 54.8831)
  line L708 (112.157, 54.8831) -> (112.157, 53.8826)
  line L709 (112.157, 53.8826) -> (111.356, 53.8826)
  line L710 (111.356, 53.8826) -> (111.356, 50.7834)
  line L711 (111.356, 50.7834) -> (112.157, 50.7834)
  line L712 (112.157, 50.7834) -> (112.157, 44.9834)
  line L713 (112.157, 44.9834) -> (111.356, 44.9834)
  line L714 (111.356, 44.9834) -> (111.356, 41.8828)
  line L715 (111.356, 41.8828) -> (112.157, 41.8828)
  line L716 (112.157, 41.8828) -> (112.157, 40.8838)
  line L717 (112.157, 40.8838) -> (126.157, 40.8838)
  line L718 (126.157, 40.8838) -> (126.157, 41.8828)
  line L719 (126.157, 41.8828) -> (126.956, 41.8828)
  line L720 (126.956, 41.8828) -> (126.956, 44.9834)
  line L721 (126.956, 44.9834) -> (126.157, 44.9834)
  line L722 (126.157, 44.9834) -> (126.157, 50.7834)
  line L723 (126.157, 50.7834) -> (126.956, 50.7834)
  line L724 (126.956, 50.7834) -> (126.956, 53.8826)
  line L725 (126.956, 53.8826) -> (126.157, 53.8826)
  line L726 (126.157, 53.8826) -> (126.157, 54.8831)
  line L727 (126.157, 54.8831) -> (112.157, 54.8831)
  line L728 (131.207, 54.8831) -> (131.207, 53.8826)
  line L729 (131.207, 53.8826) -> (130.406, 53.8826)
  line L730 (130.406, 53.8826) -> (130.406, 50.7834)
  line L731 (130.406, 50.7834) -> (131.207, 50.7834)
  line L732 (131.207, 50.7834) -> (131.207, 44.9834)
  line L733 (131.207, 44.9834) -> (130.406, 44.9834)
  line L734 (130.406, 44.9834) -> (130.406, 41.8828)
  line L735 (130.406, 41.8828) -> (131.207, 41.8828)
  line L736 (131.207, 41.8828) -> (131.207, 40.8838)
  line L737 (131.207, 40.8838) -> (145.207, 40.8838)
  line L738 (145.207, 40.8838) -> (145.207, 41.8828)
  line L739 (145.207, 41.8828) -> (146.006, 41.8828)
  line L740 (146.006, 41.8828) -> (146.006, 44.9834)
  line L741 (146.006, 44.9834) -> (145.207, 44.9834)
  line L742 (145.207, 44.9834) -> (145.207, 50.7834)
  line L743 (145.207, 50.7834) -> (146.006, 50.7834)
  line L744 (146.006, 50.7834) -> (146.006, 53.8826)
  line L745 (146.006, 53.8826) -> (145.207, 53.8826)
  line L746 (145.207, 53.8826) -> (145.207, 54.8831)
  line L747 (145.207, 54.8831) -> (131.207, 54.8831)
  line L748 (150.257, 54.8831) -> (150.257, 53.8826)
  line L749 (150.257, 53.8826) -> (149.456, 53.8826)
  line L750 (149.456, 53.8826) -> (149.456, 50.7834)
  line L751 (149.456, 50.7834) -> (150.257, 50.7834)
  line L752 (150.257, 50.7834) -> (150.257, 44.9834)
  line L753 (150.257, 44.9834) -> (149.456, 44.9834)
  line L754 (149.456, 44.9834) -> (149.456, 41.8828)
  line L755 (149.456, 41.8828) -> (150.257, 41.8828)
  line L756 (150.257, 41.8828) -> (150.257, 40.8838)
  line L757 (150.257, 40.8838) -> (164.257, 40.8838)
  line L758 (164.257, 40.8838) -> (164.257, 41.8828)
  line L759 (164.257, 41.8828) -> (165.056, 41.8828)
  line L760 (165.056, 41.8828) -> (165.056, 44.9834)
  line L761 (165.056, 44.9834) -> (164.257, 44.9834)
  line L762 (164.257, 44.9834) -> (164.257, 50.7834)
  line L763 (164.257, 50.7834) -> (165.056, 50.7834)
  line L764 (165.056, 50.7834) -> (165.056, 53.8826)
  line L765 (165.056, 53.8826) -> (164.257, 53.8826)
  line L766 (164.257, 53.8826) -> (164.257, 54.8831)
  line L767 (164.257, 54.8831) -> (150.257, 54.8831)
  line L768 (169.307, 54.8831) -> (169.307, 53.8826)
  line L769 (169.307, 53.8826) -> (168.506, 53.8826)
  line L770 (168.506, 53.8826) -> (168.506, 50.7834)
  line L771 (168.506, 50.7834) -> (169.307, 50.7834)
  line L772 (169.307, 50.7834) -> (169.307, 44.9834)
  line L773 (169.307, 44.9834) -> (168.506, 44.9834)
  line L774 (168.506, 44.9834) -> (168.506, 41.8828)
  line L775 (168.506, 41.8828) -> (169.307, 41.8828)
  line L776 (169.307, 41.8828) -> (169.307, 40.8838)
  line L777 (169.307, 40.8838) -> (183.307, 40.8838)
  line L778 (183.307, 40.8838) -> (183.307, 41.8828)
  line L779 (183.307, 41.8828) -> (184.106, 41.8828)
  line L780 (184.106, 41.8828) -> (184.106, 44.9834)
  line L781 (184.106, 44.9834) -> (183.307, 44.9834)
  line L782 (183.307, 44.9834) -> (183.307, 50.7834)
  line L783 (183.307, 50.7834) -> (184.106, 50.7834)
  line L784 (184.106, 50.7834) -> (184.106, 53.8826)
  line L785 (184.106, 53.8826) -> (183.307, 53.8826)
  line L786 (183.307, 53.8826) -> (183.307, 54.8831)
  line L787 (183.307, 54.8831) -> (169.307, 54.8831)
  line L788 (188.357, 54.8831) -> (188.357, 53.8826)
  line L789 (188.357, 53.8826) -> (187.556, 53.8826)
  line L790 (187.556, 53.8826) -> (187.556, 50.7834)
  line L791 (187.556, 50.7834) -> (188.357, 50.7834)
  line L792 (188.357, 50.7834) -> (188.357, 44.9834)
  line L793 (188.357, 44.9834) -> (187.556, 44.9834)
  line L794 (187.556, 44.9834) -> (187.556, 41.8828)
  line L795 (187.556, 41.8828) -> (188.357, 41.8828)
  line L796 (188.357, 41.8828) -> (188.357, 40.8838)
  line L797 (188.357, 40.8838) -> (202.357, 40.8838)
  line L798 (202.357, 40.8838) -> (202.357, 41.8828)
  line L799 (202.357, 41.8828) -> (203.156, 41.8828)
  line L800 (203.156, 41.8828) -> (203.156, 44.9834)
  line L801 (203.156, 44.9834) -> (202.357, 44.9834)
  line L802 (202.357, 44.9834) -> (202.357, 50.7834)
  line L803 (202.357, 50.7834) -> (203.156, 50.7834)
  line L804 (203.156, 50.7834) -> (203.156, 53.8826)
  line L805 (203.156, 53.8826) -> (202.357, 53.8826)
  line L806 (202.357, 53.8826) -> (202.357, 54.8831)
  line L807 (202.357, 54.8831) -> (188.357, 54.8831)
  line L808 (207.407, 54.8831) -> (207.407, 53.8826)
  line L809 (207.407, 53.8826) -> (206.606, 53.8826)
  line L810 (206.606, 53.8826) -> (206.606, 50.7834)
  line L811 (206.606, 50.7834) -> (207.407, 50.7834)
  line L812 (207.407, 50.7834) -> (207.407, 44.9834)
  line L813 (207.407, 44.9834) -> (206.606, 44.9834)
  line L814 (206.606, 44.9834) -> (206.606, 41.8828)
  line L815 (206.606, 41.8828) -> (207.407, 41.8828)
  line L816 (207.407, 41.8828) -> (207.407, 40.8838)
  line L817 (207.407, 40.8838) -> (221.407, 40.8838)
  line L818 (221.407, 40.8838) -> (221.407, 41.8828)
  line L819 (221.407, 41.8828) -> (222.206, 41.8828)
  line L820 (222.206, 41.8828) -> (222.206, 44.9834)
  line L821 (222.206, 44.9834) -> (221.407, 44.9834)
  line L822 (221.407, 44.9834) -> (221.407, 50.7834)
  line L823 (221.407, 50.7834) -> (222.206, 50.7834)
  line L824 (222.206, 50.7834) -> (222.206, 53.8826)
  line L825 (222.206, 53.8826) -> (221.407, 53.8826)
  line L826 (221.407, 53.8826) -> (221.407, 54.8831)
  line L827 (221.407, 54.8831) -> (207.407, 54.8831)
  line L828 (226.457, 54.8831) -> (226.457, 53.8826)
  line L829 (226.457, 53.8826) -> (225.656, 53.8826)
  line L830 (225.656, 53.8826) -> (225.656, 50.7834)
  line L831 (225.656, 50.7834) -> (226.457, 50.7834)
  line L832 (226.457, 50.7834) -> (226.457, 44.9834)
  line L833 (226.457, 44.9834) -> (225.656, 44.9834)
  line L834 (225.656, 44.9834) -> (225.656, 41.8828)
  line L835 (225.656, 41.8828) -> (226.457, 41.8828)
  line L836 (226.457, 41.8828) -> (226.457, 40.8838)
  line L837 (226.457, 40.8838) -> (240.457, 40.8838)
  line L838 (240.457, 40.8838) -> (240.457, 41.8828)
  line L839 (240.457, 41.8828) -> (241.256, 41.8828)
  line L840 (241.256, 41.8828) -> (241.256, 44.9834)
  line L841 (241.256, 44.9834) -> (240.457, 44.9834)
  line L842 (240.457, 44.9834) -> (240.457, 50.7834)
  line L843 (240.457, 50.7834) -> (241.256, 50.7834)
  line L844 (241.256, 50.7834) -> (241.256, 53.8826)
  line L845 (241.256, 53.8826) -> (240.457, 53.8826)
  line L846 (240.457, 53.8826) -> (240.457, 54.8831)
  line L847 (240.457, 54.8831) -> (226.457, 54.8831)
  line L848 (7.3822, 73.9331) -> (7.3822, 72.9326)
  line L849 (7.3822, 72.9326) -> (6.5815, 72.9326)
  line L850 (6.5815, 72.9326) -> (6.5815, 69.8334)
  line L851 (6.5815, 69.8334) -> (7.3822, 69.8334)
  line L852 (7.3822, 69.8334) -> (7.3822, 64.0334)
  line L853 (7.3822, 64.0334) -> (6.5815, 64.0334)
  line L854 (6.5815, 64.0334) -> (6.5815, 60.9328)
  line L855 (6.5815, 60.9328) -> (7.3822, 60.9328)
  line L856 (7.3822, 60.9328) -> (7.3822, 59.9338)
  line L857 (7.3822, 59.9338) -> (21.3817, 59.9338)
  line L858 (21.3817, 59.9338) -> (21.3817, 60.9328)
  line L859 (21.3817, 60.9328) -> (22.1809, 60.9328)
  line L860 (22.1809, 60.9328) -> (22.1809, 64.0334)
  line L861 (22.1809, 64.0334) -> (21.3817, 64.0334)
  line L862 (21.3817, 64.0334) -> (21.3817, 69.8334)
  line L863 (21.3817, 69.8334) -> (22.1809, 69.8334)
  line L864 (22.1809, 69.8334) -> (22.1809, 72.9326)
  line L865 (22.1809, 72.9326) -> (21.3817, 72.9326)
  line L866 (21.3817, 72.9326) -> (21.3817, 73.9331)
  line L867 (21.3817, 73.9331) -> (7.3822, 73.9331)
  line L868 (31.1947, 73.9331) -> (31.1947, 72.9326)
  line L869 (31.1947, 72.9326) -> (30.394, 72.9326)
  line L870 (30.394, 72.9326) -> (30.394, 69.8334)
  line L871 (30.394, 69.8334) -> (31.1947, 69.8334)
  line L872 (31.1947, 69.8334) -> (31.1947, 64.0334)
  line L873 (31.1947, 64.0334) -> (30.394, 64.0334)
  line L874 (30.394, 64.0334) -> (30.394, 60.9328)
  line L875 (30.394, 60.9328) -> (31.1947, 60.9328)
  line L876 (31.1947, 60.9328) -> (31.1947, 59.9338)
  line L877 (31.1947, 59.9338) -> (45.194, 59.9338)
  line L878 (45.194, 59.9338) -> (45.194, 60.9328)
  line L879 (45.194, 60.9328) -> (45.9948, 60.9328)
  line L880 (45.9948, 60.9328) -> (45.9948, 64.0334)
  line L881 (45.9948, 64.0334) -> (45.194, 64.0334)
  line L882 (45.194, 64.0334) -> (45.194, 69.8334)
  line L883 (45.194, 69.8334) -> (45.9948, 69.8334)
  line L884 (45.9948, 69.8334) -> (45.9948, 72.9326)
  line L885 (45.9948, 72.9326) -> (45.194, 72.9326)
  line L886 (45.194, 72.9326) -> (45.194, 73.9331)
  line L887 (45.194, 73.9331) -> (31.1947, 73.9331)
  line L888 (50.2447, 73.9331) -> (50.2447, 72.9326)
  line L889 (50.2447, 72.9326) -> (49.4439, 72.9326)
  line L890 (49.4439, 72.9326) -> (49.4439, 69.8334)
  line L891 (49.4439, 69.8334) -> (50.2447, 69.8334)
  line L892 (50.2447, 69.8334) -> (50.2447, 64.0334)
  line L893 (50.2447, 64.0334) -> (49.4439, 64.0334)
  line L894 (49.4439, 64.0334) -> (49.4439, 60.9328)
  line L895 (49.4439, 60.9328) -> (50.2447, 60.9328)
  line L896 (50.2447, 60.9328) -> (50.2447, 59.9338)
  line L897 (50.2447, 59.9338) -> (64.244, 59.9338)
  line L898 (64.244, 59.9338) -> (64.244, 60.9328)
  line L899 (64.244, 60.9328) -> (65.0448, 60.9328)
  line L900 (65.0448, 60.9328) -> (65.0448, 64.0334)
  line L901 (65.0448, 64.0334) -> (64.244, 64.0334)
  line L902 (64.244, 64.0334) -> (64.244, 69.8334)
  line L903 (64.244, 69.8334) -> (65.0448, 69.8334)
  line L904 (65.0448, 69.8334) -> (65.0448, 72.9326)
  line L905 (65.0448, 72.9326) -> (64.244, 72.9326)
  line L906 (64.244, 72.9326) -> (64.244, 73.9331)
  line L907 (64.244, 73.9331) -> (50.2447, 73.9331)
  line L908 (69.2947, 73.9331) -> (69.2947, 72.9326)
  line L909 (69.2947, 72.9326) -> (68.4939, 72.9326)
  line L910 (68.4939, 72.9326) -> (68.4939, 69.8334)
  line L911 (68.4939, 69.8334) -> (69.2947, 69.8334)
  line L912 (69.2947, 69.8334) -> (69.2947, 64.0334)
  line L913 (69.2947, 64.0334) -> (68.4939, 64.0334)
  line L914 (68.4939, 64.0334) -> (68.4939, 60.9328)
  line L915 (68.4939, 60.9328) -> (69.2947, 60.9328)
  line L916 (69.2947, 60.9328) -> (69.2947, 59.9338)
  line L917 (69.2947, 59.9338) -> (83.294, 59.9338)
  line L918 (83.294, 59.9338) -> (83.294, 60.9328)
  line L919 (83.294, 60.9328) -> (84.0948, 60.9328)
  line L920 (84.0948, 60.9328) -> (84.0948, 64.0334)
  line L921 (84.0948, 64.0334) -> (83.294, 64.0334)
  line L922 (83.294, 64.0334) -> (83.294, 69.8334)
  line L923 (83.294, 69.8334) -> (84.0948, 69.8334)
  line L924 (84.0948, 69.8334) -> (84.0948, 72.9326)
  line L925 (84.0948, 72.9326) -> (83.294, 72.9326)
  line L926 (83.294, 72.9326) -> (83.294, 73.9331)
  line L927 (83.294, 73.9331) -> (69.2947, 73.9331)
  line L928 (88.3447, 73.9331) -> (88.3447, 72.9326)
  line L929 (88.3447, 72.9326) -> (87.5439, 72.9326)
  line L930 (87.5439, 72.9326) -> (87.5439, 69.8334)
  line L931 (87.5439, 69.8334) -> (88.3447, 69.8334)
  line L932 (88.3447, 69.8334) -> (88.3447, 64.0334)
  line L933 (88.3447, 64.0334) -> (87.5439, 64.0334)
  line L934 (87.5439, 64.0334) -> (87.5439, 60.9328)
  line L935 (87.5439, 60.9328) -> (88.3447, 60.9328)
  line L936 (88.3447, 60.9328) -> (88.3447, 59.9338)
  line L937 (88.3447, 59.9338) -> (102.344, 59.9338)
  line L938 (102.344, 59.9338) -> (102.344, 60.9328)
  line L939 (102.344, 60.9328) -> (103.145, 60.9328)
  line L940 (103.145, 60.9328) -> (103.145, 64.0334)
  line L941 (103.145, 64.0334) -> (102.344, 64.0334)
  line L942 (102.344, 64.0334) -> (102.344, 69.8334)
  line L943 (102.344, 69.8334) -> (103.145, 69.8334)
  line L944 (103.145, 69.8334) -> (103.145, 72.9326)
  line L945 (103.145, 72.9326) -> (102.344, 72.9326)
  line L946 (102.344, 72.9326) -> (102.344, 73.9331)
  line L947 (102.344, 73.9331) -> (88.3447, 73.9331)
  line L948 (107.395, 73.9331) -> (107.395, 72.9326)
  line L949 (107.395, 72.9326) -> (106.594, 72.9326)
  line L950 (106.594, 72.9326) -> (106.594, 69.8334)